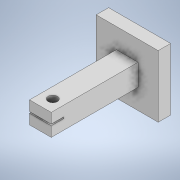
# Autodesk Inventor part: linear polariser
Saved by Autodesk Inventor 2021 (Build 250183000, 183)
## iProperties
Created: 2021-06-12
Part Number: linear polariser
Material: Generic
Document SubType Name: Modeling
Designer: user
Density: 1 g/cm^3
Appearance: Default
Author: user
Autodesk Inventor part; units mm, degrees
ref_plane "YZ Plane" through (0, 0, 0) normal (1, 0, 0) x (0, 1, 0)
ref_plane "XZ Plane" through (0, 0, 0) normal (0, 1, 0) x (-1, 0, 0)
ref_plane "XY Plane" through (0, 0, 0) normal (0, 0, 1) x (1, 0, 0)
sketch "Sketch1" plane through (0, 0, 0) normal (0, 0, 1) x (1, 0, 0)
  line L0 (-46.6309, 64.3185) -> (53.3691, 64.3185)
  line L1 (53.3691, 64.3185) -> (53.3691, -35.6815)
  line L2 (53.3691, -35.6815) -> (-46.6309, -35.6815)
  line L3 (-46.6309, -35.6815) -> (-46.6309, 64.3185)
  point P0 (0, 0)
  dimension "d0" = 100
  dimension "d1" = 100
  constraints: 8 end point, 2 parallel, 1 horizontal, 1 perpendicular
  measures "d0" distance of L0.start L0.end
  measures "d1" distance of L2.end L0.start
extrude "Extrusion1" add sketch "Sketch1" along normal blind 20
sketch "Sketch2" plane through (0, 0, 20) normal (0, 0, 1) x (1, 0, 0)
  line L0 (-14.1309, 31.8185) -> (20.8691, 31.8185)
  line L1 (20.8691, 31.8185) -> (20.8691, 15.5685)
  line L2 (20.8691, 15.5685) -> (-14.1309, 15.5685)
  line L3 (-14.1309, 15.5685) -> (-14.1309, 31.8185)
  line L4 (-14.1309, 15.5685) -> (20.8691, 15.5685)
  line L5 (20.8691, 15.5685) -> (20.8691, 13.0685)
  line L6 (20.8691, 13.0685) -> (-14.1309, 13.0685)
  line L7 (-14.1309, 13.0685) -> (-14.1309, 15.5685)
  line L8 (-14.1309, 13.0685) -> (20.8691, 13.0685)
  line L9 (20.8691, 13.0685) -> (20.8691, -3.1815)
  line L10 (20.8691, -3.1815) -> (-14.1309, -3.1815)
  line L11 (-14.1309, -3.1815) -> (-14.1309, 13.0685)
  line L12 (53.3691, 64.3185) -> (-46.6309, 64.3185) projected
  line L13 (-46.6309, -35.6815) -> (53.3691, -35.6815) projected
  line L14 (53.3691, -35.6815) -> (53.3691, 64.3185) projected
  line L15 (-46.6309, 64.3185) -> (-46.6309, -35.6815) projected
  point P0 (0, 0)
  dimension "d4" = 2.5
  dimension "d5" = 16.25
  dimension "d6" = 16.25
  dimension "d7" = 32.5
  dimension "d8" = 32.5
  dimension "d9" = 32.5
  dimension "d10" = 32.5
  dimension "d11" = 48.75
  constraints: 24 end point, 6 parallel, 4 point on line, 3 horizontal, 3 perpendicular
  measures "d4" distance between parallel lines of L6 L4
  measures "d5" distance between parallel lines of L2 L0
  measures "d6" distance between parallel lines of L8 L10
  measures "d7" distance between parallel lines of L12 L0
  measures "d8" distance between parallel lines of L13 L10
  measures "d9" distance between parallel lines of L14 L1
  measures "d10" distance between parallel lines of L15 L3
  measures "d11" distance between parallel lines of L12 L4
extrude "Extrusion2" add sketch "Sketch2" along normal blind 140 contours L0 L1 L2 L3
sketch "Sketch3" plane through (-14.1309, 15.5685, 20) normal (0, -1, 0) x (1, 0, 0)
  circle A0 centre (17.5, 120) radius 7.5
  line L0 (-32.5, 0) -> (67.5, 0) projected
  line L1 (35, 0) -> (35, 140) projected
  point P0 (14.1309, -20)
  dimension "d14" = 120
  dimension "d15" = 15
  dimension "d16" = 17.5
  constraints: 1 centre point
  measures "d14" distance from line of L0 A0.centre
  measures "d15" diameter of A0
  measures "d16" distance from line of L1 A0.centre
extrude "Extrusion3" cut sketch "Sketch3" against normal blind 150
sketch "Sketch4" plane through (0, 0, 20) normal (0, 0, 1) x (1, 0, 0)
  point P0 (0, 0)
sketch "Sketch5" plane through (0, 0, 20) normal (0, 0, 1) x (1, 0, 0)
  line L0 (-14.1309, 15.6081) -> (20.8691, 15.6081)
  line L1 (20.8691, 15.6081) -> (20.8691, 13.1081)
  line L2 (20.8691, 13.1081) -> (-14.1309, 13.1081)
  line L3 (-14.1309, 13.1081) -> (-14.1309, 15.6081)
  line L4 (-14.1309, 31.8185) -> (-14.1309, 15.5685) projected
  point P0 (0, 0)
  dimension "d19" = 35
  dimension "d20" = 2.5
  dimension "d21" = 0
  constraints: 8 end point, 2 parallel, 1 horizontal, 1 perpendicular
  measures "d19" distance of L1.end L2.end
  measures "d20" distance of L2.end L0.start
  measures "d21" distance from line of L4 L0.start
extrude "Extrusion4" add sketch "Sketch5" along normal blind 120
sketch "Sketch6" plane through (-14.1309, 13.1081, 20) normal (0, -1, 0) x (1, 0, 0)
  circle A0 centre (17.9369, 120) radius 12.75
  line L0 (-32.5, 0) -> (67.5, 0) projected
  point P0 (14.1309, -20)
  dimension "d24" = 120
  dimension "d25" = 25.5
  constraints: 1 centre point
  measures "d24" distance from line of L0 A0.centre
  measures "d25" diameter of A0
extrude "Extrusion5" cut sketch "Sketch6" against normal blind 2.5
sketch "Sketch7" plane through (0, 0, 20) normal (0, 0, 1) x (1, 0, 0)
  line L0 (-14.1309, 15.5685) -> (-14.1309, 13.1081) projected
  line L1 (-14.1309, 13.1081) -> (20.8691, 13.1081)
  line L2 (20.8691, 13.1081) -> (20.8691, -3.1419)
  line L3 (20.8691, -3.1419) -> (-14.1309, -3.1419)
  line L4 (-14.1309, -3.1419) -> (-14.1309, 13.1081)
  point P0 (0, 0)
  dimension "d28" = 16.25
  dimension "d29" = 35
  constraints: 8 end point, 2 parallel, 1 horizontal, 1 perpendicular
  measures "d28" distance of L3.end L0.end
  measures "d29" distance of L2.end L3.end
extrude "Extrusion6" add sketch "Sketch7" along normal blind 140
sketch "Sketch8" plane through (-14.1309, -3.1419, 20) normal (0, -1, 0) x (1, 0, 0)
  circle A0 centre (17.5, 120) radius 7.5
  line L0 (35, 0) -> (35, 140) projected
  line L1 (-32.5, 0) -> (67.5, 0) projected
  point P0 (14.1309, -20)
  dimension "d33" = 17.5
  dimension "d34" = 15
  dimension "d35" = 120
  constraints: 1 centre point
  measures "d33" distance from line of L0 A0.centre
  measures "d34" diameter of A0
  measures "d35" distance from line of L1 A0.centre
extrude "Extrusion7" cut sketch "Sketch8" against normal blind 16.25
equation "\"d1\" = d0"
equation "\"d6\" = d5"
equation "\"d8\" = d7"
equation "\"d10\" = d9"
body "Solid1"
